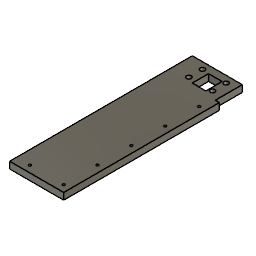
right engine cover lol (Autodesk Fusion 360 design; units mm, degrees)
Autodesk Fusion 360 part; units mm, degrees
sketch "Szkic1" plane through (0, 0, 0) normal (0, 0, 1) x (1, 0, 0)
  line L0 (29, -30) -> (29, 10)
  line L1 (-31, -30) -> (29, -30)
  line L2 (-31, 10) -> (-31, -30)
  line L3 (29, 10) -> (-31, 10)
  line L4 (-10, -1) -> (10, -1)
  line L5 (-10, -25) -> (-10, -1)
  line L6 (10, -25) -> (-10, -25)
  line L7 (10, -1) -> (10, -25)
  circle A0 centre (15, -20) radius 2
  circle A1 centre (15, 0) radius 2
  circle A2 centre (-20, 0) radius 2
  circle A3 centre (-20, -20) radius 2
  line L8 (29, 10) -> (29, -30)
  line L9 (29, -30) -> (35, -30)
  line L10 (35, -30) -> (35, 10)
  line L11 (35, 10) -> (29, 10)
  line L12 (-31, 10) -> (-31, -30)
  line L13 (-31, -30) -> (-45, -30)
  line L14 (-45, -30) -> (-45, 10)
  line L15 (-45, 10) -> (-31, 10)
  line L16 (35, -30) -> (35, -260)
  line L17 (-45, -30) -> (-45, -260)
  line L18 (-45, -260) -> (35, -260)
  circle A4 centre (-20, 0) radius 3.5
  circle A5 centre (-20, -20) radius 3.5
  circle A6 centre (15, -20) radius 3.5
  circle A7 centre (15, 0) radius 3.5
  dimension "d1" = 4
  dimension "d2" = 4
  dimension "d3" = 4
  dimension "d4" = 6
  dimension "d5" = 14
  dimension "d6" = 230
  dimension "d7" = 230
  dimension "d8" = 7
  dimension "d9" = 7
  dimension "d10" = 7
  dimension "d11" = 7
  constraint perpendicular L4 L7
  constraint parallel L4 L6
  constraint parallel L5 L7
  constraint perpendicular L1 L2
  constraint parallel L0 L2
  constraint parallel L1 L3
  constraint perpendicular L8 L9
  constraint parallel L8 L10
  constraint parallel L9 L11
  constraint perpendicular L12 L13
  constraint parallel L12 L14
  constraint parallel L13 L15
  constraint perpendicular L9 L16
  constraint perpendicular L13 L17
  constraint concentric A2 A4
  constraint concentric A3 A5
  constraint concentric A0 A6
  constraint concentric A1 A7
  measures "d1" diameter of A3
  measures "d2" diameter of A2
  measures "d3" diameter of A1
  measures "d4" distance of L0.end L10.end
  measures "d5" distance of L2.start L14.end
  measures "d6" distance of L9.end L16.end
  measures "d7" distance of L13.end L17.end
  measures "d8" diameter of A4
  measures "d9" diameter of A5
  measures "d10" diameter of A6
  measures "d11" diameter of A7
extrude "Wyciągnięcie proste1" add sketch "Szkic1" against normal blind 10 contours L0 L1 L2 L3 L8 L12 | L1 L9 L13 L16 L17 L18 | L2 L12 L13 L14 L15 | A4 | A5 | A6 | A7
extrude "Wyciągnięcie proste2" cut sketch "Szkic1" against normal blind 5 contours A4 | A5 | A6 | A7
sketch "Szkic2" plane through (0, 0, -10) normal (0, 0, -1) x (1, 0, 0)
  circle A0 centre (-20, 20) radius 2
  line L0 (10, 1) -> (-10, 1)
  line L1 (-10, 1) -> (-10, 25)
  line L2 (-10, 25) -> (10, 25)
  line L3 (10, 25) -> (10, 1)
  circle A1 centre (15, 20) radius 2
  circle A2 centre (15, 0) radius 2
  circle A3 centre (-20, 0) radius 2
  line L4 (-45, 260) -> (-45, -10)
  line L5 (-45, -10) -> (29, -10)
  line L6 (29, -10) -> (29, 30)
  line L7 (29, 30) -> (35, 30)
  line L8 (35, 30) -> (35, 260)
  line L9 (35, 260) -> (-45, 260)
  circle A4 centre (25, 250) radius 1.75
  circle A5 centre (-25, 250) radius 1.75
  circle A6 centre (25, 200) radius 1.75
  circle A7 centre (25, 150) radius 1.75
  circle A8 centre (25, 100) radius 1.75
  circle A9 centre (25, 50) radius 1.75
  circle A10 centre (25, 50) radius 3.5
  circle A11 centre (25, 100) radius 3.5
  circle A12 centre (25, 150) radius 3.5
  circle A13 centre (25, 200) radius 3.5
  circle A14 centre (25, 250) radius 3.5
  circle A15 centre (-25, 250) radius 3.5
  dimension "d16" = 3.5
  dimension "d17" = 3.5
  dimension "d18" = 3.5
  dimension "d19" = 3.5
  dimension "d20" = 3.5
  dimension "d21" = 3.5
  dimension "d22" = 7
  dimension "d23" = 7
  dimension "d24" = 7
  dimension "d25" = 7
  dimension "d26" = 7
  dimension "d27" = 7
  constraint concentric A9 A10
  constraint concentric A8 A11
  constraint concentric A7 A12
  constraint concentric A6 A13
  constraint concentric A4 A14
  constraint concentric A5 A15
  measures "d16" diameter of A4
  measures "d17" diameter of A5
  measures "d18" diameter of A6
  measures "d19" diameter of A7
  measures "d20" diameter of A8
  measures "d21" diameter of A9
  measures "d22" diameter of A10
  measures "d23" diameter of A11
  measures "d24" diameter of A12
  measures "d25" diameter of A13
  measures "d26" diameter of A14
  measures "d27" diameter of A15
extrude "Wyciągnięcie proste3" cut sketch "Szkic2" against normal blind 5 contours A10 | A11 | A12 | A13 | A14 | A15
extrude "Wyciągnięcie proste4" cut 6 faces at (-25.7416, -250.3286, -10) (24.2584, -250.3286, -10) (23.7552, -199.6385, -10) (23.7552, -149.6385, -10) (25.3956, -99.1189, -10) (25.1298, -50.5687, -10) along direction (0, 0, 1) blind 10
